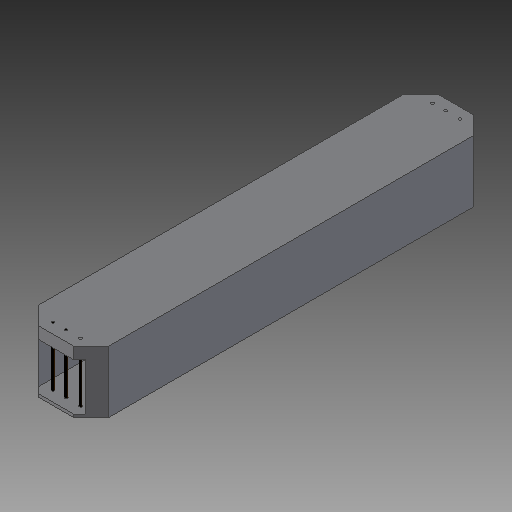
# Autodesk Inventor part: 1112_Magnet Brick Housing_V1
Saved by Autodesk Inventor 2020 (Build 240168000, 168)
## iProperties
Created: 2019-10-13
Part Number: 1112_Magnet Brick Housing_V1
Material: Acetal Resin, White
Document SubType Name: Modeling
Designer: RFLab
Density: 1.425 g/cm^3
Appearance: Smooth - White
Mass: 1479 g
Surface Area: 2133.9 cm^2
Volume: 1037.89 cm^3
Author: RFLab
Autodesk Inventor part; units mm, degrees
ref_plane "YZ Plane" through (0, 0, 0) normal (1, 0, 0) x (0, 1, 0)
ref_plane "XZ Plane" through (0, 0, 0) normal (0, 1, 0) x (-1, 0, 0)
ref_plane "XY Plane" through (0, 0, 0) normal (0, 0, 1) x (1, 0, 0)
sketch "Sketch1" plane through (0, 0, 0) normal (0, 0, 1) x (1, 0, 0)
  line L0 (-25.4, -25.4) -> (25.4, -25.4)
  line L1 (25.4, -25.4) -> (25.4, 25.4)
  line L2 (25.4, 25.4) -> (-25.4, 25.4)
  line L3 (-25.4, 25.4) -> (-25.4, -25.4)
  line L4 (-25.4, -25.4) -> (25.4, 25.4) construction
  line L5 (25.4, -25.4) -> (-25.4, 25.4) construction
  line L6 (-38.1, 38.1) -> (38.1, 38.1)
  line L7 (38.1, 38.1) -> (38.1, -38.1)
  line L8 (38.1, -38.1) -> (-38.1, -38.1)
  line L9 (-38.1, -38.1) -> (-38.1, 38.1)
  line L10 (-38.1, -28.575) -> (38.1, -28.575)
  point P0 (0, 0)
  dimension "d0" = 50.8
  dimension "d1" = 50.8
  dimension "d2" = 12.7
  dimension "d3" = 3.175
  constraints: 22 end point, 4 parallel, 3 perpendicular, 2 midpoint, 2 point on line, 1 horizontal, 3 other
  measures "d0" distance of L2.end L1.end
  measures "d1" distance of L1.end L0.end
  measures "d2" distance between parallel lines of L2 L6
  measures "d3" distance between parallel lines of L0 L10
extrude "Extrusion1" add sketch "Sketch1" along normal mid plane 431.8 contours L6 L7 L10 L9
sketch "Sketch2" plane through (-38.1, 38.1, 215.9) normal (0, 1, 0) x (1, 0, 0)
  line L0 (0, 431.8) -> (0, 0) construction
  line L1 (76.2, 0) -> (0, 0) projected
  line L2 (76.2, 431.8) -> (76.2, 0) construction
  line L3 (0, 431.8) -> (76.2, 431.8) construction
  line L4 (0, 0) -> (0, 431.8) construction
  line L5 (0, 412.75) -> (19.05, 431.8)
  line L6 (0, 412.75) -> (26.9408, 412.75) construction
  line L7 (63.5, 431.8) -> (12.7, 431.8) construction
  line L8 (38.1, 431.8) -> (38.1, 0) construction
  line L9 (0, 0) -> (76.2, 0) projected
  line L10 (0, 412.75) -> (0, 431.8)
  line L11 (0, 431.8) -> (19.05, 431.8)
  line L12 (0, 431.8) -> (76.2, 431.8) projected
  line L13 (76.2, 412.75) -> (57.15, 431.8)
  line L14 (76.2, 412.75) -> (76.2, 431.8)
  line L15 (76.2, 431.8) -> (57.15, 431.8)
  line L16 (0, 215.9) -> (38.1, 215.9) construction
  line L17 (0, 19.05) -> (19.05, 0)
  line L18 (0, 19.05) -> (26.9408, 19.05) construction
  line L19 (0, 19.05) -> (0, 0)
  line L20 (0, 0) -> (19.05, 0)
  line L21 (76.2, 19.05) -> (76.2, 0)
  line L22 (76.2, 0) -> (57.15, 0)
  line L23 (76.2, 19.05) -> (57.15, 0)
  point P0 (63.5, 0)
  point P1 (12.7, 0)
  dimension "d6" = 45
  dimension "d7" = 19.05
  constraints: 32 end point, 9 symmetric about line, 3 midpoint, 2 collinear, 2 horizontal, 2 point on line, 1 equal length
  measures "d6" angle of L6 L5
  measures "d7" distance of L0.start L5.start
extrude "Extrusion2" cut sketch "Sketch2" against normal through all
sketch "Sketch3" plane through (-19.05, 38.1, -215.9) normal (0, 1, 0) x (1, 0, 0)
  line L0 (-6.35, -419.1) -> (44.45, -419.1) construction
  line L1 (44.45, -419.1) -> (44.45, -12.7) construction
  line L2 (44.45, -12.7) -> (-6.35, -12.7) construction
  line L3 (-6.35, -12.7) -> (-6.35, -419.1) construction
  line L4 (-19.05, -19.05) -> (-19.05, -412.75) construction
  line L5 (0, 0) -> (38.1, 0) construction
  line L6 (38.1, -431.8) -> (0, -431.8) construction
  line L7 (-19.05, -412.75) -> (-19.05, -19.05) construction
  line L8 (-19.05, -215.9) -> (19.05, -215.9) construction
  line L9 (38.1, 0) -> (0, 0) construction
  line L10 (19.05, 0) -> (19.05, -215.9) construction
  circle A0 centre (4.8101, -11.2) radius 1.5
  circle A1 centre (34.45, -11.2) radius 1.5
  circle A2 centre (19.05, -11.2) radius 1.5
  point P0 (-6.35, -215.9)
  point P1 (19.05, -12.7)
  point P2 (19.05, 0)
  dimension "d10" = 50.8
  dimension "d11" = 406.4
  dimension "d12" = 3
  dimension "d13" = 3
  dimension "d14" = 3
  dimension "d15" = 11.1601
  dimension "d16" = 10
  constraints: 12 end point, 5 midpoint, 3 centre point, 3 tangent, 2 horizontal, 2 parallel, 2 perpendicular, 1 horizontal alignment, 1 point on line, 1 vertical alignment
  measures "d10" distance of L2.end L1.end
  measures "d11" distance of L1.end L0.end
  measures "d12" diameter of A0
  measures "d13" diameter of A1
  measures "d14" diameter of A2
  measures "d15" distance from line of L3 A0.centre
  measures "d16" distance from line of L1 A1.centre
extrude "Extrusion3" add sketch "Sketch3" against normal up to surface (63.5 mm away) separate body
mirror "Mirror1" about plane through (0, 0, 0) normal (0, 0, 1) of "Extrusion3" bodies 2
body "Solid1"
body "Solid2"
